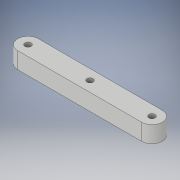
# Autodesk Inventor part: Hebel_KLemme_Hebel
Saved by Autodesk Inventor 2018 (Build 220112000, 112)
## iProperties
Created: 2018-02-02
Part Number: Hebel_KLemme_Hebel
Material: Generisch
Document SubType Name: Modeling
Designer: Julian
Density: 1 g/cm^3
Appearance: Vorgabe
Author: Julian
Autodesk Inventor part; units mm, degrees
ref_plane "YZ Plane" through (0, 0, 0) normal (1, 0, 0) x (0, 1, 0)
ref_plane "XZ Plane" through (0, 0, 0) normal (0, 1, 0) x (-1, 0, 0)
ref_plane "XY Plane" through (0, 0, 0) normal (0, 0, 1) x (1, 0, 0)
sketch "Skizze1" plane through (0, 0, 0) normal (0, 0, 1) x (1, 0, 0)
  line L0 (2.5, 0) -> (32.5, 0)
  line L1 (35, 2.5) -> (35, 2.5)
  line L2 (32.5, 5) -> (2.5, 5)
  line L3 (0, 2.5) -> (0, 2.5)
  arc A0 (2.5, 5) -> (0, 2.5) centre (2.5, 2.5) ccw
  arc A1 (0, 2.5) -> (2.5, 0) centre (2.5, 2.5) ccw
  arc A2 (35, 2.5) -> (32.5, 5) centre (32.5, 2.5) ccw
  arc A3 (32.5, 0) -> (35, 2.5) centre (32.5, 2.5) ccw
  point P0 (0, 0)
  point P1 (35, 5)
  point P2 (35, 0)
  point P3 (0, 5)
  dimension "d0" = 35
  dimension "d1" = 5
  dimension "d14" = 2.5
  constraints: 8 end point, 8 point on circle, 8 point on line, 8 tangent, 4 centre point, 3 equal radius, 2 parallel, 1 horizontal, 1 perpendicular
  measures "d0" distance of point (0, 5) point (35, 5)
  measures "d1" distance of point (35, 0) point (35, 5)
  measures "d14" radius of A0
extrude "Extrusion1" add sketch "Skizze1" along normal blind 4
sketch "Skizze2" plane through (0, 0, 4) normal (0, 0, 1) x (1, 0, 0)
  line L0 (0, 0) -> (32.5, 0) projected
  line L1 (0, 0) -> (2.5, 0)
  line L2 (2.5, 0) -> (0, 0)
  line L3 (2.5, 0) -> (2.5, 2.5)
  circle A0 centre (2.5, 2.5) radius 0.75
  line L4 (35, 0) -> (32.5, 0)
  line L5 (32.5, 0) -> (32.5, 2.5)
  circle A1 centre (32.5, 2.5) radius 0.75
  line L6 (0, 0) -> (17.5, 0)
  line L7 (17.5, 0) -> (17.5, 2.5)
  circle A2 centre (17.5, 2.5) radius 0.75
  dimension "d4" = 2.5
  dimension "d5" = 2.5
  dimension "d6" = 2.5
  dimension "d7" = 1.5
  dimension "d8" = 2.5
  dimension "d9" = 17.5
  dimension "d10" = 1.5
  dimension "d11" = 1.5
  constraints: 15 end point, 3 centre point, 3 coincident, 2 perpendicular, 2 point on line, 1 collinear, 1 vertical
  measures "d4" distance of L0.start L1.end
  measures "d5" distance of L1.end L0.start
  measures "d6" distance of L1.end L3.end
  measures "d7" diameter of A0
  measures "d8" distance of L4.start L0.end
  measures "d9" distance of L0.start L6.end
  measures "d10" diameter of A2
  measures "d11" diameter of A1
extrude "Extrusion2" cut sketch "Skizze2" against normal blind 10
